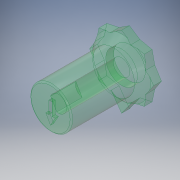
# Autodesk Inventor part: potcap
Saved by Autodesk Inventor 2017 SP1 (Build 210196100, 196)
## iProperties
Created: 2016-12-24
Part Number: potcap
Material: Generic
Document SubType Name: Modeling
Designer: wsh32
Density: 1 g/cm^3
Appearance: Clear - Green 1
Author: wsh32
Autodesk Inventor part; units mm, degrees
ref_plane "YZ Plane" through (0, 0, 0) normal (1, 0, 0) x (0, 1, 0)
ref_plane "XZ Plane" through (0, 0, 0) normal (0, 1, 0) x (-1, 0, 0)
ref_plane "XY Plane" through (0, 0, 0) normal (0, 0, 1) x (1, 0, 0)
sketch "Sketch1" plane through (0, 0, 0) normal (0, 0, 1) x (1, 0, 0)
  circle A0 centre (0, 0) radius 2.9845
  circle A1 centre (0, 0) radius 8.382
  circle A2 centre (0, 0) radius 3.302
  dimension "d0" = 5.969
  dimension "d2" = 0.3175
  dimension "d5" = 5.08
  constraints: 3 centre point, 1 coincident
  measures "d0" diameter of A0
  measures "d2" radial gap between concentric circles of A0 A2
  measures "d5" radial gap between concentric circles of A1 A2
extrude "Extrusion1" add sketch "Sketch1" along normal blind 25.4 contours A1
sketch "Sketch2" plane through (0, 0, 25.4) normal (0, 0, 1) x (1, 0, 0)
  circle A0 centre (0, 0) radius 8.382 projected
extrude "Extrusion2" add sketch "Sketch2" along normal blind 3.175
sketch "Sketch3" plane through (0, 0, 28.575) normal (0, 0, 1) x (1, 0, 0)
  line L0 (0.635, -2.54) -> (-0.635, -2.54)
  line L1 (-0.635, -2.54) -> (-0.635, 2.54)
  line L2 (-0.635, 2.54) -> (0.635, 2.54)
  line L3 (0.635, 2.54) -> (0.635, -2.54)
  line L4 (0.635, -2.54) -> (-0.635, 2.54) construction
  line L5 (-0.635, -2.54) -> (0.635, 2.54) construction
  line L6 (0, 2.54) -> (0, -2.54) construction
  line L7 (-1.905, -2.54) -> (1.905, -2.54)
  line L8 (1.905, -2.54) -> (0, -5.9267)
  line L9 (0, -5.9267) -> (-1.905, -2.54)
  point P0 (0, 0)
  dimension "d8" = 5.08
  dimension "d10" = 1.27
  dimension "d11" = 3.81
  dimension "d45" = 3.3867
  constraints: 20 end point, 4 midpoint, 2 horizontal, 2 parallel, 1 collinear, 1 perpendicular, 1 point on line, 1 symmetric about line
  measures "d8" distance of L2.end L0.start
  measures "d10" distance of L1.end L2.end
  measures "d11" distance of L7.start L7.end
  measures "d45" distance from line of L8.end L7
extrude "Extrusion3" cut sketch "Sketch3" against normal blind 1.27
chamfer "Chamfer1" distance 0.508 angle 45 1 edges at (-8.382, 0, 28.575)
sketch "Sketch6" plane through (0, 0, 25.4) normal (0, 0, -1) x (-1, 0, 0)
  circle A0 centre (0, 0) radius 3.302 projected
  line L0 (0.6206, 3.2432) -> (3.1189, -1.0842) construction
  line L1 (3.1189, 1.0842) -> (0.6206, -3.2432)
  line L2 (0, 0) -> (3.302, 0) construction
  circle A1 centre (0, 0) radius 3.302 construction
  line L3 (0, 0) -> (2.8596, -1.651) construction
  line L4 (0, 0) -> (2.8596, 1.651) construction
  line L5 (-1.3144, 4.3273) -> (-3.8128, 0) construction
  arc A2 (0.6206, -3.2432) -> (3.1189, 1.0842) centre (0, 0) ccw
  dimension "d24" = 60
  dimension "d26" = 5.461
  constraints: 12 end point, 4 point on circle, 2 equal length, 2 symmetric about line, 1 centre point, 1 horizontal, 1 parallel, 1 point on line, 11 other
  measures "d24" angle of L3 L4
  measures "d26" distance between parallel lines of L5 L1
extrude "Extrusion6" add sketch "Sketch6" along normal blind 10.16 contours A0 L1 picked at (1.6947, -1.725)
sketch "Sketch8" plane through (0, 0, 0) normal (0, 0, -1) x (-1, 0, 0)
  circle A0 centre (0, 0) radius 6.35
  line L0 (-5.8725, 9.0515) -> (0, 12.8615)
  line L1 (0, 12.8615) -> (5.8725, 9.0515)
  line L2 (0, 0) -> (0, 12.8615) construction
  circle A1 centre (0, 0) radius 10.7896
  circle A2 centre (0, 0) radius 3.302 construction
  circle A3 centre (0, 0) radius 8.382 construction
  line L3 (-10.5528, 2.2479) -> (-9.0944, 9.0944)
  line L4 (-9.0944, 9.0944) -> (-2.2479, 10.5528)
  line L5 (0, 0) -> (-9.0944, 9.0944) construction
  circle A4 centre (0, 0) radius 10.7896
  line L6 (-9.0515, -5.8725) -> (-12.8615, 0)
  line L7 (-12.8615, 0) -> (-9.0515, 5.8725)
  line L8 (0, 0) -> (-12.8615, 0) construction
  circle A5 centre (0, 0) radius 10.7896
  line L9 (-2.2479, -10.5528) -> (-9.0944, -9.0944)
  line L10 (-9.0944, -9.0944) -> (-10.5528, -2.2479)
  line L11 (0, 0) -> (-9.0944, -9.0944) construction
  circle A6 centre (0, 0) radius 10.7896
  line L12 (5.8725, -9.0515) -> (0, -12.8615)
  line L13 (0, -12.8615) -> (-5.8725, -9.0515)
  line L14 (0, 0) -> (0, -12.8615) construction
  circle A7 centre (0, 0) radius 10.7896
  line L15 (10.5528, -2.2479) -> (9.0944, -9.0944)
  line L16 (9.0944, -9.0944) -> (2.2479, -10.5528)
  line L17 (0, 0) -> (9.0944, -9.0944) construction
  circle A8 centre (0, 0) radius 10.7896
  line L18 (9.0515, 5.8725) -> (12.8615, 0)
  line L19 (12.8615, 0) -> (9.0515, -5.8725)
  line L20 (0, 0) -> (12.8615, 0) construction
  circle A9 centre (0, 0) radius 10.7896
  line L21 (2.2479, 10.5528) -> (9.0944, 9.0944)
  line L22 (9.0944, 9.0944) -> (10.5528, 2.2479)
  line L23 (0, 0) -> (9.0944, 9.0944) construction
  circle A10 centre (0, 0) radius 10.7896
  dimension "d31" = 12.7
  dimension "d32" = 3.81
  dimension "d34" = 5.08
  dimension "d35" = 4.4396
  dimension "d38" = 360
  constraints: 48 end point, 16 point on circle, 9 centre point, 9 coincident, 1 tangent, 1 vertical, 74 other
  measures "d31" diameter of A0
  measures "d32" vertical distance of L0.end L1.end
  measures "d34" radial gap between concentric circles of A3 A2
  measures "d35" radial gap between concentric circles of A0 A1
extrude "Extrusion8" add sketch "Sketch8" along normal blind 3.175
chamfer "Chamfer2" distance 3.175 angle 45 1 edges at (-8.382, 0, 0)
sketch "Sketch9" plane through (0, 0, -3.175) normal (0, 0, -1) x (-1, 0, 0)
  circle A0 centre (0, 0) radius 6.35 construction
  line L0 (10.1372, 4.199) -> (9.0944, 9.0944) construction
  line L1 (9.0944, 9.0944) -> (4.199, 10.1372) construction
  line L2 (4.199, 10.1372) -> (0, 12.8615) construction
  line L3 (0, 12.8615) -> (-4.199, 10.1372) construction
  line L4 (-4.199, 10.1372) -> (-9.0944, 9.0944) construction
  line L5 (-9.0944, 9.0944) -> (-10.1372, 4.199) construction
  line L6 (-10.1372, 4.199) -> (-12.8615, 0) construction
  line L7 (-12.8615, 0) -> (-10.1372, -4.199) construction
  line L8 (-10.1372, -4.199) -> (-9.0944, -9.0944) construction
  line L9 (-9.0944, -9.0944) -> (-4.199, -10.1372) construction
  line L10 (-4.199, -10.1372) -> (0, -12.8615) construction
  line L11 (0, -12.8615) -> (4.199, -10.1372) construction
  line L12 (4.199, -10.1372) -> (9.0944, -9.0944) construction
  line L13 (9.0944, -9.0944) -> (10.1372, -4.199) construction
  line L14 (10.1372, -4.199) -> (12.8615, 0) construction
  line L15 (12.8615, 0) -> (10.1372, 4.199) construction
  line L16 (4.199, -10.1372) -> (0, -16.0365)
  line L17 (-4.199, -10.1372) -> (0, -12.8615) construction
  line L18 (0, -16.0365) -> (-4.199, -10.1372)
  line L19 (0, 0) -> (0, -16.0365) construction
  line L20 (4.199, -10.1372) -> (9.0944, -9.0944) projected
  line L21 (-9.0944, -9.0944) -> (-4.199, -10.1372) projected
  line L22 (4.199, -10.1372) -> (-4.199, -10.1372)
  dimension "d46" = 3.175
  constraints: 8 end point, 1 horizontal, 1 vertical
  measures "d46" distance of L16.end L10.end
extrude "Extrusion9" add sketch "Sketch9" against normal up to surface (3.175 mm away)
equation "\"d11\" = 3 * d10"
equation "\"d45\" = 0.666667 * d8"
body "Solid1"
